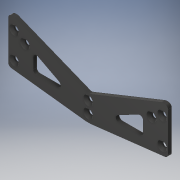
# Autodesk Inventor part: Plaque arriere
Saved by Autodesk Inventor 2019 (Build 230136000, 136)
## iProperties
Created: 2019-07-29
Part Number: Plaque arriere
Material: Résine phénolique
Document SubType Name: Modeling
Designer: Sébastien DI MERCURIO
Mass: 9.71824 g
Surface Area: 69.74 cm^2
Volume: 7.0422 cm^3
Density: 1.38 g/cm^3
Appearance: Lisse - Noir
Author: Sébastien DI MERCURIO
Autodesk Inventor part; units mm, degrees
ref_plane "YZ Plane" through (0, 0, 0) normal (1, 0, 0) x (0, 1, 0)
ref_plane "XZ Plane" through (0, 0, 0) normal (0, 1, 0) x (-1, 0, 0)
ref_plane "XY Plane" through (0, 0, 0) normal (0, 0, 1) x (1, 0, 0)
sketch "Esquisse1" plane through (0, 0, 0) normal (0, 0, 1) x (1, 0, 0)
  line L0 (0, 0) -> (97, 0)
  line L1 (97, 0) -> (97, 33)
  line L2 (97, 33) -> (0, 33)
  line L3 (0, 33) -> (0, 0)
  dimension "d0" = 33
  dimension "d1" = 97
  constraints: 8 end point, 2 parallel, 1 horizontal, 1 perpendicular
  measures "d0" distance of L2.end L0.start
  measures "d1" distance of L1.end L2.end
extrude "Extrusion1" add sketch "Esquisse1" along normal blind 2.2
sketch "Esquisse2" plane through (0, 0, 2.2) normal (0, 0, 1) x (1, 0, 0)
  line L0 (48.5, 54.7001) -> (48.5, -34.6149)
  line L1 (97, 0) -> (97, 33) construction
  line L2 (0, 33) -> (0, 0) construction
  circle A0 centre (48.5, 4.5) radius 1.5
  circle A1 centre (48.5, 11.5) radius 1.5
  circle A2 centre (3.5, 26) radius 1.5
  circle A3 centre (3.5, 10) radius 1.5
  circle A4 centre (10, 22) radius 1.5
  line L3 (0, 0) -> (97, 0) projected
  line L4 (97, 33) -> (0, 33) projected
  circle A5 centre (93.5, 26) radius 1.5
  circle A6 centre (93.5, 10) radius 1.5
  circle A7 centre (87, 22) radius 1.5
  dimension "d4" = 48.5
  dimension "d5" = 97
  dimension "d6" = 3
  dimension "d7" = 4.5
  dimension "d8" = 7
  dimension "d9" = 7
  dimension "d10" = 16
  dimension "d11" = 4
  dimension "d12" = 3.5
  dimension "d13" = 3.5
  dimension "d14" = 10
  constraints: 8 centre point, 4 equal radius, 3 symmetric about line, 2 end point, 2 point on line, 1 vertical, 3 other
  measures "d4" distance from line of L0 L2.end
  measures "d5" distance between parallel lines of L1 L2
  measures "d6" diameter of A2
  measures "d7" distance from line of L3 A0.centre
  measures "d8" distance of A0.centre A1.centre
  measures "d9" distance from line of L4 A2.centre
  measures "d10" distance of A3.centre A2.centre
  measures "d11" vertical distance of A4.centre A2.centre
  measures "d12" distance from line of L2 A2.centre
  measures "d13" distance from line of L2 A3.centre
  measures "d14" distance from line of L2 A4.centre
extrude "Extrusion2" cut sketch "Esquisse2" against normal through all
sketch "Esquisse3" plane through (0, 0, 2.2) normal (0, 0, 1) x (1, 0, 0)
  line L0 (48.5, 41.6615) -> (48.5, -20.3357)
  line L1 (97, 0) -> (97, 33) projected
  line L2 (0, 33) -> (0, 0) projected
  line L3 (3.5, 33) -> (48.5, 15)
  line L4 (48.5, 33) -> (3.5, 33)
  line L5 (97, 33) -> (0, 33) projected
  line L6 (0, 5.5) -> (47, 0)
  line L7 (0, 0) -> (97, 0) projected
  line L8 (47, 0) -> (0, 0)
  line L9 (0, 0) -> (0, 5.5)
  line L10 (0, 33) -> (0, 0) projected
  line L11 (15, 21) -> (15, 9)
  line L12 (15, 9) -> (38, 9)
  line L13 (38, 9) -> (15, 21)
  line L14 (82, 21) -> (82, 9)
  line L15 (82, 9) -> (59, 9)
  line L16 (59, 9) -> (82, 21)
  line L17 (93.5, 33) -> (48.5, 15)
  line L18 (48.5, 33) -> (93.5, 33)
  line L19 (97, 5.5) -> (50, 0)
  line L20 (50, 0) -> (97, 0)
  line L21 (97, 0) -> (97, 5.5)
  dimension "d17" = 97
  dimension "d18" = 48.5
  dimension "d19" = 45
  dimension "d20" = 5.5
  dimension "d21" = 47
  dimension "d22" = 18
  dimension "d23" = 15
  dimension "d24" = 12
  dimension "d25" = 23
  dimension "d26" = 15
  dimension "d27" = 9
  constraints: 34 end point, 6 symmetric about line, 4 point on line, 2 collinear, 2 vertical, 1 horizontal, 1 perpendicular
  measures "d17" distance between parallel lines of L1 L2
  measures "d18" distance between parallel lines of L2 L0
  measures "d19" distance of L4.start L3.start
  measures "d20" distance of L2.end L6.start
  measures "d21" distance of L2.end L6.end
  measures "d22" distance of L3.end L4.start
  measures "d23" distance from line of L7 L3.end
  measures "d24" distance of L11.start L11.end
  measures "d25" distance of L11.end L12.end
  measures "d26" distance between parallel lines of L2 L11
  measures "d27" distance between parallel lines of L7 L12
extrude "Extrusion3" cut sketch "Esquisse3" against normal through all contours L5 L17 L0 | L0 L3 L4 | L7 L2 L6 | L19 L1 L7 | L13 L12 L11 | L14 L15 L16
fillet "Congé1" radius 2 15 edges at (0, 33, 1.1) (97, 33, 1.1) (97, 5.5, 1.1) (0, 5.5, 1.1) (47, 0, 1.1) (50, 0, 1.1) (48.5, 15, 1.1) (3.5, 33, 1.1) (93.5, 33, 1.1) (59, 9, 1.1) (82, 9, 1.1) (82, 21, 1.1) (38, 9, 1.1) (15, 9, 1.1) (15, 21, 1.1)
chamfer "Chanfrein1" distance 1.5 angle 45 8 edges at (2, 26, 2.2) (8.5, 22, 2.2) (2, 10, 2.2) (47, 11.5, 2.2) (47, 4.5, 2.2) (92, 10, 2.2) (85.5, 22, 2.2) (92, 26, 2.2)
equation "\"d4\" = 0.5 * d5"
equation "\"d13\" = d12"
equation "\"d18\" = 0.5 * d17"
